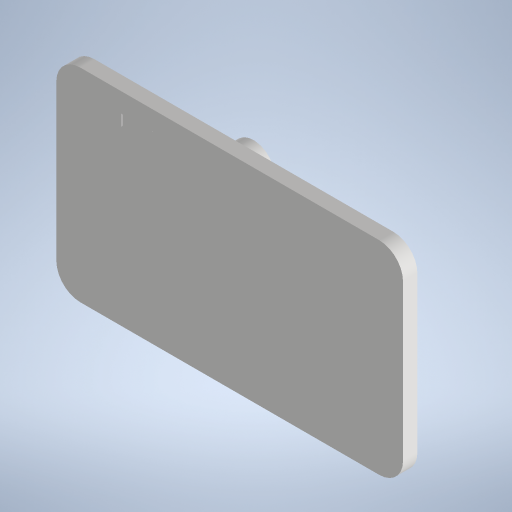
# Autodesk Inventor part: 버튼 스위치
Saved by Autodesk Inventor 2023 (Build 270158000, 158)
## iProperties
Created: 2022-06-24
Part Number: 버튼 스위치
Material: 일반
Document SubType Name: Modeling
Designer: user
Density: 1 g/cm^3
Appearance: 기본값
Author: user
Autodesk Inventor part; units mm, degrees
ref_plane "XZ Plane" through (0, 0, 0) normal (0, 1, 0) x (-1, 0, 0)
ref_plane "XY Plane" through (0, 0, 0) normal (0, 0, 1) x (1, 0, 0)
sketch "스케치1" plane through (0, 0, 0) normal (0, 0, 1) x (1, 0, 0)
  line L0 (-36.25, 21.25) -> (36.25, 21.25)
  line L1 (36.25, 21.25) -> (36.25, -21.25)
  line L2 (36.25, -21.25) -> (-36.25, -21.25)
  line L3 (-36.25, -21.25) -> (-36.25, 21.25)
  line L4 (-36.25, 21.25) -> (36.25, -21.25) construction
  line L5 (36.25, 21.25) -> (-36.25, -21.25) construction
  point P0 (0, 0)
  dimension "d0" = 72.5
  dimension "d1" = 42.5
  constraints: 12 end point, 2 midpoint, 2 parallel, 1 horizontal, 1 perpendicular
  measures "d0" distance of L1.end L2.end
  measures "d1" distance of L0.end L1.end
extrude "돌출1" add sketch "스케치1" along normal blind 3
sketch "스케치2" plane through (0, 0, 0) normal (0, 0, -1) x (-1, 0, 0)
  line L0 (2.25, 19.075) -> (-2.25, 19.075)
  line L1 (-2.25, 19.075) -> (-2.25, 14.575)
  line L2 (-2.25, 14.575) -> (2.25, 14.575)
  line L3 (2.25, 14.575) -> (2.25, 19.075)
  line L4 (2.25, 19.075) -> (-2.25, 14.575) construction
  line L5 (-2.25, 19.075) -> (2.25, 14.575) construction
  line L6 (0, 0) -> (9.8887, 0)
  line L7 (2.25, -19.075) -> (-2.25, -19.075)
  line L8 (-2.25, -19.075) -> (-2.25, -14.575)
  line L9 (-2.25, -14.575) -> (2.25, -14.575)
  line L10 (2.25, -14.575) -> (2.25, -19.075)
  line L11 (2.25, -19.075) -> (-2.25, -14.575) construction
  line L12 (-2.25, -19.075) -> (2.25, -14.575) construction
  line L13 (36.25, -21.25) -> (-36.25, -21.25) projected
  line L14 (36.25, 21.25) -> (36.25, -21.25) projected
  line L15 (-36.25, 21.25) -> (36.25, 21.25) projected
  line L16 (-36.25, -21.25) -> (-36.25, 21.25) projected
  circle A0 centre (0, 16.825) radius 4.425
  circle A1 centre (0, -16.825) radius 4.425
  point P0 (0, 21.25)
  point P1 (0, -21.25)
  dimension "d4" = 4.5
  dimension "d5" = 4.5
  dimension "d6" = 16.825
  constraints: 26 end point, 5 symmetric about line, 4 midpoint, 3 vertical alignment, 2 coincident, 2 horizontal, 2 parallel, 1 perpendicular, 4 other
  measures "d4" distance of L0.start L0.end
  measures "d5" distance of L2.end L0.start
  measures "d6" distance of L6.start point (0, 16.825)
extrude "돌출2" add sketch "스케치2" along normal blind 2 contours A0 | A1
fillet "모깎기1" radius 5 4 edges at (-36.25, 21.25, 1.5) (36.25, 21.25, 1.5) (36.25, -21.25, 1.5) (-36.25, -21.25, 1.5)
sketch "스케치5" plane through (0, 0, 3) normal (0, 0, 1) x (1, 0, 0)
  line L0 (-22.5, 15) -> (22.5, 15)
  line L1 (22.5, 15) -> (22.5, 17)
  line L2 (22.5, 17) -> (-22.5, 17)
  line L3 (-22.5, 17) -> (-22.5, 15)
  line L4 (-22.5, 15) -> (22.5, 17) construction
  line L5 (22.5, 15) -> (-22.5, 17) construction
  point P0 (0, 0)
  point P1 (0, 16)
  dimension "d18" = 2
  dimension "d19" = 45
  dimension "d20" = 16
  constraints: 12 end point, 2 midpoint, 2 parallel, 1 horizontal, 1 perpendicular, 1 vertical alignment
  measures "d18" distance of L2.end L0.start
  measures "d19" distance of L1.end L2.end
  measures "d20" distance of point (0, 0) point (0, 16)
extrude "돌출4" cut sketch "스케치5" against normal blind 0.2
chamfer "모따기1" distance 0.2 angle 45 4 edges at (0, 17, 3) (-22.5, 16, 3) (0, 15, 3) (22.5, 16, 3)
ref_plane "작업 평면1" through (22.8, 0, 0) normal (1, 0, 0) x (0, 1, 0)
sketch "스케치6" plane through (22.8, 0, 0) normal (1, 0, 0) x (0, 1, 0)
  line L0 (0, 0) -> (0, -4)
  circle A0 centre (0, -4) radius 4
  line L1 (0, 0) -> (5, 0)
  line L2 (-16.25, 0) -> (16.25, 0) construction
  line L3 (5, 0) -> (3.9024, -4.878)
  line L4 (0, 0) -> (-5, 0)
  line L5 (-5, 0) -> (-3.6851, -5.5556)
  circle A1 centre (0, -4) radius 2
  dimension "d27" = 8
  dimension "d28" = 10
  dimension "d29" = 4
  dimension "d30" = 4
  constraints: 10 end point, 2 centre point, 2 coincident, 2 point on circle, 1 point on line, 1 symmetric about line, 1 tangent, 1 vertical
  measures "d27" diameter of A0
  measures "d28" distance of L4.end L1.end
  measures "d29" diameter of A1
  measures "d30" distance of L0.start L0.end
extrude "돌출5" add sketch "스케치6" against normal blind 3 contours A0 L5 | A0 L1 L3 | A0 L5 L4 picked at (-3.2164, -4.7153)
mirror "미러1" about plane through (0, 0, 0) normal (1, 0, 0) of "돌출5"
fillet "모깎기2" radius 0.3 2 edges at (22.8, -2, -4) (-22.8, -2, -4)
sketch "스케치7" plane through (0, 0, 0) normal (0, 0, -1) x (-1, 0, 0)
  line L0 (2.25, 19.075) -> (-2.25, 19.075) projected
  line L1 (-2.25, 19.075) -> (-2.25, 14.575) projected
  line L2 (-2.25, 14.575) -> (2.25, 14.575) projected
  line L3 (2.25, 14.575) -> (2.25, 19.075) projected
  line L4 (2.25, -19.075) -> (2.25, -14.575) projected
  line L5 (2.25, -14.575) -> (-2.25, -14.575) projected
  line L6 (-2.25, -14.575) -> (-2.25, -19.075) projected
  line L7 (-2.25, -19.075) -> (2.25, -19.075) projected
  point P0 (0, 0)
extrude "돌출6" add sketch "스케치7" along normal blind 0.5
sketch "스케치8" plane through (-19.8, -5, 0) normal (1, 0, 0) x (0, 0, -1)
  arc A0 (5.5556, 1.3149) -> (4.878, 8.9024) centre (4, 5) ccw projected
  line L0 (4.878, 8.9024) -> (8, 8.9024)
  line L1 (8, 8.9024) -> (8, 1.1545)
  line L2 (8, 1.1545) -> (4.878, 1.1545)
  line L3 (4.878, 1.1545) -> (4.878, 8.9024)
  line L4 (0, 0) -> (5.5556, 1.3149) projected
  point P0 (0, 5)
  point P1 (8, 5)
  constraints: 8 end point, 2 parallel, 1 horizontal, 1 perpendicular, 1 point on line, 1 tangent
extrude "돌출7" add sketch "스케치8" against normal blind 3 contours A0 L1 L2 L4 | A0 L0 L1
chamfer "모따기2" distance 1 angle 45 2 edges at (-21.3, 3.9024, -8) (-21.3, -3.8455, -8)
mirror "미러2" about plane through (0, 0, 0) normal (1, 0, 0) of "돌출7", "모따기2"
